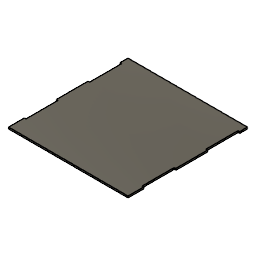
Tafel (Autodesk Fusion 360 archive; units mm, degrees)
design "tafel plaat"
part number: 2026-04-23-08-51-58-937
Autodesk Fusion 360 part; units mm, degrees
sketch "Sketch1" plane through (0, 0, 0) normal (0, 0, 1) x (1, 0, 0)
  line L0 (-73.0553, -57.6886) -> (226.9447, -57.6886)
  line L1 (226.9447, 242.3114) -> (-73.0553, 242.3114)
  line L2 (-73.0553, 222.3114) -> (-69.0553, 222.3114)
  line L3 (-69.0553, 222.3114) -> (-69.0553, 142.3114)
  line L4 (-69.0553, 142.3114) -> (-73.0553, 142.3114)
  line L5 (-73.0553, 242.3114) -> (-73.0553, 222.3114)
  line L6 (-73.0553, -17.6886) -> (-69.0553, -17.6886)
  line L7 (-69.0553, -17.6886) -> (-69.0553, 62.3114)
  line L8 (-69.0553, 62.3114) -> (-73.0553, 62.3114)
  line L9 (-73.0553, 142.3114) -> (-73.0553, 62.3114)
  line L10 (-73.0553, -17.6886) -> (-73.0553, -57.6886)
  line L11 (226.9447, 222.3114) -> (222.9447, 222.3114)
  line L12 (222.9447, 222.3114) -> (222.9447, 142.3114)
  line L13 (222.9447, 142.3114) -> (226.9447, 142.3114)
  line L14 (226.9447, 62.3114) -> (222.9447, 62.3114)
  line L15 (222.9447, 62.3114) -> (222.9447, -17.6886)
  line L16 (222.9447, -17.6886) -> (226.9447, -17.6886)
  line L17 (226.9447, -17.6886) -> (226.9447, -57.6886)
  line L18 (226.9447, 142.3114) -> (226.9447, 62.3114)
  line L19 (226.9447, 242.3114) -> (226.9447, 222.3114)
  dimension "d1" = 300
  dimension "d2" = 300
  dimension "d3" = 20
  dimension "d4" = 4
  dimension "d5" = 80
  dimension "d6" = 80
  dimension "d7" = 80
  dimension "d8" = 4
  dimension "d9" = 4
  dimension "d10" = 80
  dimension "d11" = 20
  dimension "d12" = 80
  dimension "d13" = 80
  constraint horizontal L0
  constraint horizontal L1
  constraint horizontal L2
  constraint vertical L3
  constraint horizontal L4
  constraint perpendicular L2 L5
  constraint horizontal L6
  constraint vertical L7
  constraint horizontal L8
  constraint perpendicular L4 L9
  constraint perpendicular L0 L10
  constraint horizontal L11
  constraint vertical L12
  constraint horizontal L13
  constraint horizontal L14
  constraint vertical L15
  constraint horizontal L16
  constraint perpendicular L0 L17
  constraint perpendicular L14 L18
  constraint perpendicular L11 L19
  measures "d1" distance of L0.start L0.end
  measures "d2" distance of L0.start L1.end
  measures "d3" distance of L1.end L2.start
  measures "d4" distance of L2.start L2.end
  measures "d5" distance of L2.start L4.end
  measures "d6" distance of L6.end L7.end
  measures "d7" distance of L3.end L7.end
  measures "d8" distance of L11.start L11.end
  measures "d9" distance of L14.start L14.end
  measures "d10" distance of L11.end L12.end
  measures "d11" distance of L1.start L11.start
  measures "d12" distance of L12.end L14.end
  measures "d13" distance of L14.end L15.end
extrude "Extrude1" add sketch "Sketch1" along normal blind 4

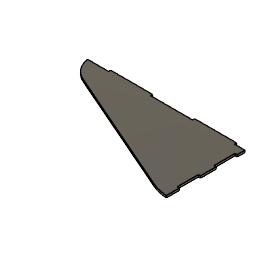
design "tafel zij"
part number: 2026-04-23-09-05-02-427
Autodesk Fusion 360 part; units mm, degrees
sketch "Sketch1" plane through (0, 0, 0) normal (0, 0, 1) x (1, 0, 0)
  line L0 (-51.5127, 19.8666) -> (-51.5127, 23.8666)
  line L1 (-51.5127, 23.8666) -> (28.4873, 23.8666)
  line L2 (28.4873, 23.8666) -> (28.4873, 19.8666)
  line L3 (-211.5127, 19.8666) -> (-211.5127, 23.8666)
  line L4 (-211.5127, 23.8666) -> (-131.5127, 23.8666)
  line L5 (-131.5127, 23.8666) -> (-131.5127, 19.8666)
  line L6 (48.4873, 4.8666) -> (44.4873, 4.8666)
  line L7 (44.4873, 4.8666) -> (44.4873, -35.1334)
  line L8 (44.4873, -35.1334) -> (48.4873, -35.1334)
  line L9 (48.4873, -65.1334) -> (44.4873, -65.1334)
  line L10 (44.4873, -65.1334) -> (44.4873, -105.1334)
  line L11 (44.4873, -105.1334) -> (48.4873, -105.1334)
  line L12 (-251.5127, 19.8666) -> (-211.5127, 19.8666)
  line L13 (-131.5127, 19.8666) -> (-51.5127, 19.8666)
  line L14 (28.4873, 19.8666) -> (48.4873, 19.8666)
  line L15 (48.4873, 4.8666) -> (48.4873, 6.5368)
  line L16 (48.4873, 6.5368) -> (48.4873, 19.8666)
  line L17 (48.4873, -35.1334) -> (48.4873, -65.1334)
  line L18 (48.4873, -105.1334) -> (48.4873, -130.1334)
  line L19 (17.9193, -122.7788) -> (-223.306, -17.2487)
  arc A0 (-251.5127, 19.8666) -> (-223.306, -17.2487) centre (-204.1197, 26.6083) ccw
  arc A1 (17.9193, -122.7788) -> (48.4873, -130.1334) centre (53.8475, -40.6527) ccw
  dimension "d1" = 300
  dimension "d2" = 150
  dimension "d3" = 4
  dimension "d4" = 4
  dimension "d5" = 80
  dimension "d6" = 80
  dimension "d7" = 20
  dimension "d8" = 80
  dimension "d9" = 4
  dimension "d10" = 4
  dimension "d11" = 40
  dimension "d12" = 40
  dimension "d13" = 30
  dimension "d14" = 15
  constraint vertical L0
  constraint horizontal L1
  constraint vertical L2
  constraint vertical L3
  constraint horizontal L4
  constraint vertical L5
  constraint horizontal L6
  constraint vertical L7
  constraint horizontal L8
  constraint horizontal L9
  constraint vertical L10
  constraint horizontal L11
  constraint perpendicular L3 L12
  constraint perpendicular L5 L13
  constraint perpendicular L6 L15
  constraint perpendicular L14 L16
  constraint perpendicular L9 L17
  constraint perpendicular L11 L18
  constraint tangent L19 A0
  constraint tangent L19 A1
  measures "d1" distance of L12.start L14.end
  measures "d2" distance of L14.end L18.end
  measures "d3" distance of L3.start L3.end
  measures "d4" distance of L0.start L0.end
  measures "d5" distance of L3.end L4.end
  measures "d6" distance of L0.end L1.end
  measures "d7" distance of L14.end L2.end
  measures "d8" distance of L0.start L5.end
  measures "d9" distance of L9.start L9.end
  measures "d10" distance of L6.start L6.end
  measures "d11" distance of L6.end L7.end
  measures "d12" distance of L9.end L10.end
  measures "d13" distance of L8.end L9.start
  measures "d14" distance of L14.end L6.start
extrude "Extrude1" add sketch "Sketch1" along normal blind 4
